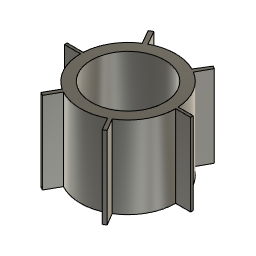
Tombo 2 v1 (Autodesk Fusion 360 design; units mm, degrees)
Autodesk Fusion 360 part; units mm, degrees
sketch "Sketch1" plane through (0, 0, 0) normal (0, 0, 1) x (1, 0, 0)
sketch "Sketch2" plane through (0, 0, 0) normal (0, 0, 1) x (1, 0, 0)
  circle A0 centre (0, 0) radius 111.6729
  line L0 (-194, 0) -> (-145, 0)
  line L1 (-144.7791, 8) -> (-194, 8)
  line L2 (-194, 8) -> (-194, 0)
  line L3 (191, 0) -> (145, 0)
  line L4 (144.7791, 8) -> (191, 8)
  line L5 (191, 8) -> (191, 0)
  line L6 (-93.2448, -168.0185) -> (-69.9873, -126.9913)
  line L7 (-103.1731, -162.3904) -> (-79.7615, -121.0913)
  line L8 (-103.1731, -162.3904) -> (-93.2448, -168.0185)
  arc A1 (-145, 0) -> (-79.7615, -121.0913) centre (0, 0) ccw
  line L9 (-102.8058, 164.3391) -> (-78.5783, 121.8624)
  line L10 (-67.6654, 128.2435) -> (-91.9168, 170.7622)
  line L11 (-91.9168, 170.7622) -> (-102.8058, 164.3391)
  arc A2 (-78.5783, 121.8624) -> (-144.7791, 8) centre (0, 0) ccw
  line L12 (65.0496, 129.5899) -> (90, 170)
  line L13 (90, 170) -> (98.2091, 164.9314)
  line L14 (98.2091, 164.9314) -> (75.4604, 123.8173)
  arc A3 (144.7791, 8) -> (75.4604, 123.8173) centre (0, 0) ccw
  arc A4 (65.0496, 129.5899) -> (-67.6654, 128.2435) centre (0, 0) ccw
  line L15 (88.714, -167.4802) -> (98.1586, -161.8134)
  line L16 (98.1586, -161.8134) -> (75.3876, -123.8617)
  line L17 (66.4486, -128.8782) -> (88.714, -167.4802)
  arc A5 (-69.9873, -126.9913) -> (66.4486, -128.8782) centre (0, 0) ccw
  arc A6 (75.3876, -123.8617) -> (145, 0) centre (0, 0) ccw
  dimension "d1" = 290
  constraint coincident A0.centre A1.centre
  constraint concentric A0 A5
  constraint horizontal L0
  constraint horizontal L1
  constraint vertical L2
  constraint horizontal L3
  constraint horizontal L4
  constraint vertical L5
  constraint perpendicular L6 L8
  constraint concentric A3 A5
  constraint coincident L0.end A3
  constraint concentric A1 A3
  constraint coincident L9.end A3
  constraint concentric A2 A3
  constraint coincident L12.start A3
  constraint perpendicular L12 L13
  constraint concentric A3 A4
  constraint coincident L16.end A5
  constraint perpendicular L15 L16
  constraint concentric A5 A6
  measures "d1" diameter of A5
extrude "Extrude1" add sketch "Sketch2" along normal blind 250
